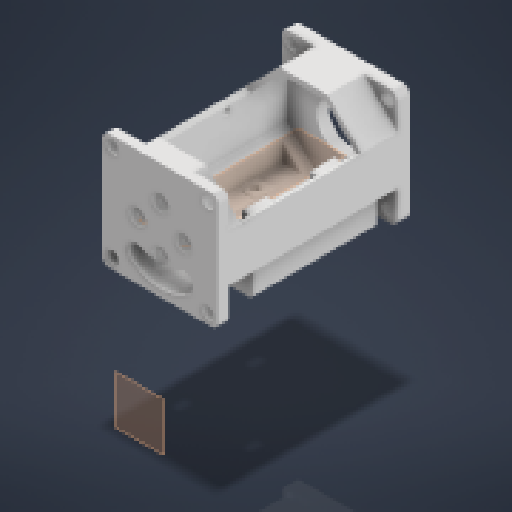
# Autodesk Inventor part: КорпусЕСК
Saved by Autodesk Inventor 2026 (Build 300175000, 175)
## iProperties
Created: 2025-08-20
Part Number: КорпусЕСК
Material: Типовые
Document SubType Name: Modeling
Designer: seraf
Density: 1 g/cm^3
Appearance: По умолчанию
Author: seraf
Autodesk Inventor part; units mm, degrees
ref_plane "YZ Plane" through (0, 0, 0) normal (1, 0, 0) x (0, 1, 0)
ref_plane "XZ Plane" through (0, 0, 0) normal (0, 1, 0) x (-1, 0, 0)
ref_plane "РабПлоскость1" through (0, 0, 25.75) normal (0, 0, 1) x (1, 0, 0)
sketch "Эскиз1" plane through (0, 0, 25.75) normal (0, 0, 1) x (1, 0, 0)
  circle A0 centre (30.5216, 91.6095) radius 2.5 projected
  circle A1 centre (10.7206, 81.3105) radius 1.5 projected
  circle A2 centre (1.2206, 71.8105) radius 1.5 projected
  circle A3 centre (-9.0784, 52.0095) radius 2.5 projected
  circle A4 centre (10.7206, 62.3105) radius 1.5 projected
  circle A5 centre (30.5216, 52.0095) radius 2.5 projected
  circle A6 centre (-9.0784, 91.6095) radius 2.5 projected
  circle A7 centre (20.2206, 71.8105) radius 1.5 projected
  arc A8 (34.7206, 92.8105) -> (31.7206, 95.8105) centre (31.7206, 92.8105) ccw projected
  line L0 (34.7206, 50.8105) -> (34.7206, 92.8105) projected
  arc A9 (31.7206, 47.8105) -> (34.7206, 50.8105) centre (31.7206, 50.8105) ccw projected
  line L1 (-10.2794, 47.8105) -> (31.7206, 47.8105) projected
  arc A10 (-13.2794, 50.8105) -> (-10.2794, 47.8105) centre (-10.2794, 50.8105) ccw projected
  line L2 (-13.2794, 92.8105) -> (-13.2794, 50.8105) projected
  arc A11 (-10.2794, 95.8105) -> (-13.2794, 92.8105) centre (-10.2794, 92.8105) ccw projected
  line L3 (31.7206, 95.8105) -> (-10.2794, 95.8105) projected
  arc A12 (-0.1228, 54.4431) -> (21.5639, 54.4431) centre (10.7206, 68.8105) ccw projected
  arc A13 (21.5639, 54.4431) -> (19.9477, 62.2015) centre (20.2206, 58.2108) ccw projected
  arc A14 (1.4934, 62.2015) -> (19.9477, 62.2015) centre (10.7206, 78.8105) ccw projected
  arc A15 (1.4934, 62.2015) -> (-0.1228, 54.4431) centre (1.2206, 58.2108) ccw projected
  point P0 (0, 0)
extrude "Выдавливание1" add sketch "Эскиз1" along normal blind 2
chamfer "Фаска1" distance 2 angle 45 4 edges at (9.2206, 62.3105, 27.75) (18.7206, 71.8105, 27.75) (9.2206, 81.3105, 27.75) (-0.2794, 71.8105, 27.75)
sketch "Эскиз2" plane through (0, 0, 25.75) normal (0, 0, -1) x (-1, 0, 0)
  line L0 (-31.7206, 95.8105) -> (10.2794, 95.8105) projected
  arc A0 (-31.7206, 95.8105) -> (-34.7206, 92.8105) centre (-31.7206, 92.8105) ccw projected
  line L1 (-34.7206, 50.8105) -> (-34.7206, 92.8105) projected
  arc A1 (-34.7206, 50.8105) -> (-31.7206, 47.8105) centre (-31.7206, 50.8105) ccw projected
  line L2 (10.2794, 47.8105) -> (-31.7206, 47.8105) projected
  arc A2 (10.2794, 47.8105) -> (13.2794, 50.8105) centre (10.2794, 50.8105) ccw projected
  line L3 (13.2794, 92.8105) -> (13.2794, 50.8105) projected
  arc A3 (13.2794, 92.8105) -> (10.2794, 95.8105) centre (10.2794, 92.8105) ccw projected
  circle A4 centre (-10.7206, 81.3105) radius 1.5 construction
  circle A5 centre (-1.2206, 71.8105) radius 1.5 construction
  circle A6 centre (-20.2206, 71.8105) radius 1.5 construction
  arc A7 (-19.9477, 62.2015) -> (-1.4934, 62.2015) centre (-10.7206, 78.8105) ccw projected
  arc A8 (0.1228, 54.4431) -> (-1.4934, 62.2015) centre (-1.2206, 58.2108) ccw projected
  arc A9 (-21.5639, 54.4431) -> (0.1228, 54.4431) centre (-10.7206, 68.8105) ccw projected
  arc A10 (-19.9477, 62.2015) -> (-21.5639, 54.4431) centre (-20.2206, 58.2108) ccw projected
  circle A11 centre (9.0784, 91.6095) radius 2.5 projected
  circle A12 centre (-30.5216, 52.0095) radius 2.5 projected
  circle A13 centre (-10.7206, 62.3105) radius 1.5 construction
  circle A14 centre (9.0784, 52.0095) radius 2.5 projected
  circle A15 centre (-30.5216, 91.6095) radius 2.5 projected
  point P0 (0, 0)
extrude "Выдавливание2" add sketch "Эскиз2" along normal blind 2
sketch "Эскиз3" plane through (0, 0, 23.75) normal (0, 0, -1) x (-1, 0, 0)
  line L0 (-31.7206, 47.8105) -> (10.2794, 47.8105) construction
  arc A0 (10.2794, 47.8105) -> (13.2794, 50.8105) centre (10.2794, 50.8105) ccw construction
  line L1 (13.2794, 50.8105) -> (13.2794, 92.8105) construction
  arc A1 (13.2794, 92.8105) -> (10.2794, 95.8105) centre (10.2794, 92.8105) ccw construction
  line L2 (10.2794, 95.8105) -> (-31.7206, 95.8105) construction
  arc A2 (-31.7206, 95.8105) -> (-34.7206, 92.8105) centre (-31.7206, 92.8105) ccw construction
  line L3 (-34.7206, 92.8105) -> (-34.7206, 50.8105) construction
  arc A3 (-34.7206, 50.8105) -> (-31.7206, 47.8105) centre (-31.7206, 50.8105) ccw construction
  circle A4 centre (-30.5216, 91.6095) radius 2.5 construction
  circle A5 centre (9.0784, 52.0095) radius 2.5 construction
  circle A6 centre (-30.5216, 52.0095) radius 2.5 construction
  circle A7 centre (9.0784, 91.6095) radius 2.5 construction
  arc A8 (-19.9477, 62.2015) -> (-21.5639, 54.4431) centre (-20.2206, 58.2108) ccw construction
  arc A9 (-19.9477, 62.2015) -> (-1.4934, 62.2015) centre (-10.7206, 78.8105) ccw construction
  arc A10 (0.1228, 54.4431) -> (-1.4934, 62.2015) centre (-1.2206, 58.2108) ccw construction
  arc A11 (-21.5639, 54.4431) -> (0.1228, 54.4431) centre (-10.7206, 68.8105) ccw construction
  line L4 (-34.7206, 71.8105) -> (-34.7206, 81.8105)
  line L5 (-34.7206, 81.8105) -> (-20.7206, 95.8105)
  line L6 (-20.7206, 95.8105) -> (-0.7206, 95.8105)
  line L7 (-0.7206, 95.8105) -> (13.2794, 81.8105)
  line L8 (13.2794, 81.8105) -> (13.2794, 71.8105)
  line L9 (-34.7206, 71.8105) -> (13.2794, 71.8105)
  line L10 (13.2794, 92.8105) -> (13.2794, 50.8105) construction
  arc A12 (10.2794, 47.8105) -> (13.2794, 50.8105) centre (10.2794, 50.8105) ccw construction
  line L11 (10.2794, 47.8105) -> (-31.7206, 47.8105) construction
  arc A13 (-34.7206, 50.8105) -> (-31.7206, 47.8105) centre (-31.7206, 50.8105) ccw construction
  line L12 (-34.7206, 50.8105) -> (-34.7206, 92.8105) construction
  circle A14 centre (-30.5216, 52.0115) radius 2.5 construction
  circle A15 centre (9.0784, 52.0115) radius 2.5 construction
  line L13 (-34.7206, 71.8105) -> (-34.7206, 61.8105)
  line L14 (-34.7206, 61.8105) -> (-20.7206, 47.8105)
  line L15 (-20.7206, 47.8105) -> (-0.7206, 47.8105)
  line L16 (-0.7206, 47.8105) -> (13.2794, 61.8105)
  line L17 (13.2794, 61.8105) -> (13.2794, 71.8105)
  line L18 (-1.7206, 50.0826) -> (-19.7206, 50.0826)
  line L19 (-19.7206, 50.0826) -> (-32.4485, 62.8105)
  line L20 (-32.4485, 62.8105) -> (-32.4485, 80.8105)
  line L21 (-32.4485, 80.8105) -> (-19.7206, 93.5384)
  line L22 (-19.7206, 93.5384) -> (-1.7206, 93.5384)
  line L23 (-1.7206, 93.5384) -> (11.0074, 80.8105)
  line L24 (11.0074, 80.8105) -> (11.0074, 62.8105)
  line L25 (11.0074, 62.8105) -> (-1.7206, 50.0826)
  point P0 (0, 0)
  point P1 (-10.7206, 64.8105)
  point P2 (-10.7206, 71.8105)
  dimension "d8" = 20
  dimension "d9" = 1
  constraints: 44 end point, 13 symmetric about line, 8 point on line, 4 centre point, 4 point on circle, 3 midpoint, 2 equal length, 2 perpendicular, 1 horizontal, 21 other
  measures "d8" distance of L5.end L6.end
  measures "d9" horizontal distance of L16.start L18.start
extrude "Выдавливание3" add sketch "Эскиз3" along normal blind 5 contours L4 L5 L6 L7 L8 L9 L24 L23 L22 L21 L20 | L9 L20 L19 L18 L25 L24 L17 L16 L15 L14 L13
sketch "Эскиз4" plane through (0, 0, 18.75) normal (0, 0, -1) x (-1, 0, 0)
  line L0 (-34.7206, 61.8105) -> (-20.7206, 47.8105) projected
  line L1 (-20.7206, 47.8105) -> (-0.7206, 47.8105) projected
  line L2 (-0.7206, 47.8105) -> (13.2794, 61.8105) projected
  line L3 (13.2794, 61.8105) -> (13.2794, 81.8105) projected
  line L4 (13.2794, 81.8105) -> (-0.7206, 95.8105) construction
  line L5 (-0.7206, 95.8105) -> (-20.7206, 95.8105) construction
  line L6 (-20.7206, 95.8105) -> (-34.7206, 81.8105) construction
  line L7 (-34.7206, 81.8105) -> (-34.7206, 61.8105) projected
  line L8 (-32.4485, 62.8105) -> (-32.4485, 80.8105) projected
  line L9 (-32.4485, 80.8105) -> (-19.7206, 93.5384) construction
  line L10 (-19.7206, 93.5384) -> (-1.7206, 93.5384) construction
  line L11 (-1.7206, 93.5384) -> (11.0074, 80.8105) construction
  line L12 (11.0074, 80.8105) -> (11.0074, 62.8105) projected
  line L13 (11.0074, 62.8105) -> (-1.7206, 50.0826) projected
  line L14 (-1.7206, 50.0826) -> (-19.7206, 50.0826) projected
  line L15 (-19.7206, 50.0826) -> (-32.4485, 62.8105) projected
  line L16 (-34.7206, 81.8105) -> (-32.4485, 80.8105)
  line L17 (13.2794, 81.8105) -> (11.0074, 80.8105)
  point P0 (0, 0)
  constraints: 4 end point
extrude "Выдавливание4" add sketch "Эскиз4" along normal blind 50
sketch "Эскиз5" plane through (0, 0, -31.25) normal (0, 0, -1) x (-1, 0, 0)
  line L0 (-34.7206, 61.8105) -> (-20.7206, 47.8105) projected
  line L1 (-20.7206, 47.8105) -> (-0.7206, 47.8105) projected
  line L2 (-0.7206, 47.8105) -> (13.2794, 61.8105) projected
  line L3 (13.2794, 61.8105) -> (13.2794, 81.8105) projected
  line L4 (13.2794, 81.8105) -> (11.0074, 80.8105) construction
  line L5 (11.0074, 80.8105) -> (11.0074, 62.8105) projected
  line L6 (11.0074, 62.8105) -> (-1.7206, 50.0826) projected
  line L7 (-1.7206, 50.0826) -> (-19.7206, 50.0826) projected
  line L8 (-19.7206, 50.0826) -> (-32.4485, 62.8105) projected
  line L9 (-32.4485, 62.8105) -> (-32.4485, 80.8105) projected
  line L10 (-32.4485, 80.8105) -> (-34.7206, 81.8105) construction
  line L11 (-34.7206, 81.8105) -> (-34.7206, 61.8105) projected
  line L12 (11.0074, 80.8105) -> (13.2794, 81.8105) construction
  line L13 (13.2794, 81.8105) -> (-0.7206, 95.8105) projected
  line L14 (-0.7206, 95.8105) -> (-20.7206, 95.8105) projected
  line L15 (-20.7206, 95.8105) -> (-34.7206, 81.8105) projected
  line L16 (-34.7206, 81.8105) -> (-32.4485, 80.8105) construction
  line L17 (-32.4485, 80.8105) -> (-19.7206, 93.5384) projected
  line L18 (-19.7206, 93.5384) -> (-1.7206, 93.5384) projected
  line L19 (-1.7206, 93.5384) -> (11.0074, 80.8105) projected
  point P0 (0, 0)
extrude "Выдавливание5" add sketch "Эскиз5" along normal blind 15
sketch "Эскиз6" plane through (0, 0, -46.25) normal (0, 0, -1) x (-1, 0, 0)
  circle A0 centre (-10.7206, 81.3105) radius 3.5 construction
  circle A1 centre (-30.5216, 91.6095) radius 2.5 projected
  circle A2 centre (9.0784, 52.0095) radius 2.5 projected
  circle A3 centre (-30.5216, 52.0095) radius 2.5 projected
  circle A4 centre (9.0784, 91.6095) radius 2.5 projected
  line L0 (-31.7206, 95.8105) -> (10.2794, 95.8105) projected
  arc A5 (13.2794, 92.8105) -> (10.2794, 95.8105) centre (10.2794, 92.8105) ccw projected
  line L1 (13.2794, 92.8105) -> (13.2794, 50.8105) projected
  arc A6 (10.2794, 47.8105) -> (13.2794, 50.8105) centre (10.2794, 50.8105) ccw projected
  line L2 (10.2794, 47.8105) -> (-31.7206, 47.8105) projected
  arc A7 (-34.7206, 50.8105) -> (-31.7206, 47.8105) centre (-31.7206, 50.8105) ccw projected
  line L3 (-34.7206, 50.8105) -> (-34.7206, 92.8105) projected
  arc A8 (-31.7206, 95.8105) -> (-34.7206, 92.8105) centre (-31.7206, 92.8105) ccw projected
  arc A9 (-8.0984, 59.9923) -> (-13.3428, 59.9923) centre (-10.7206, 62.3105) ccw construction
  arc A10 (-19.9477, 62.2015) -> (-13.3428, 59.9923) centre (-10.7206, 78.8105) ccw construction
  arc A11 (-19.9477, 62.2015) -> (-21.5639, 54.4431) centre (-20.2206, 58.2108) ccw construction
  arc A12 (-21.5639, 54.4431) -> (0.1228, 54.4431) centre (-10.7206, 68.8105) ccw construction
  arc A13 (0.1228, 54.4431) -> (-1.4934, 62.2015) centre (-1.2206, 58.2108) ccw construction
  arc A14 (-8.0984, 59.9923) -> (-1.4934, 62.2015) centre (-10.7206, 78.8105) ccw construction
  circle A15 centre (-20.2206, 71.8105) radius 3.5 construction
  circle A16 centre (-1.2206, 71.8105) radius 3.5 construction
  circle A17 centre (-10.7206, 71.8105) radius 9.5
  point P0 (0, 0)
  dimension "d16" = 19
  constraints: 2 point on circle, 1 centre point
  measures "d16" diameter of A17
extrude "Выдавливание6" add sketch "Эскиз6" along normal blind 5
ref_plane "РабПлоскость3" through (1.7206, 70.0826, 23.75) normal (0, 1, 0) x (1, 0, 0)
sketch "Эскиз8" plane through (1.7206, 70.0826, 23.75) normal (0, 1, 0) x (1, 0, 0)
  line L0 (30, -4) -> (33, -4) projected
  line L1 (-12, 75) -> (-15, 75) projected
  line L2 (-15, 75) -> (33, 75) construction
  line L3 (33, 75) -> (33, -4) construction
  line L4 (33, -4) -> (-15, -4) construction
  line L5 (-15, -4) -> (-15, 75) construction
  circle A0 centre (23.75, 50) radius 1.5 construction
  line L6 (23.75, 50) -> (23.75, 19.5) construction
  line L7 (23.75, 19.5) -> (-5.75, 19.5) construction
  line L8 (-5.75, 19.5) -> (-5.75, 50) construction
  circle A1 centre (-5.75, 50) radius 1.5
  circle A2 centre (23.75, 19.5) radius 1.5
  circle A3 centre (-5.75, 19.5) radius 1.5
  circle A4 centre (-5.75, 50) radius 4
  circle A5 centre (-5.75, 19.5) radius 4
  circle A6 centre (23.75, 19.5) radius 4
  point P0 (-1.7206, 23.75)
  dimension "d22" = 3
  dimension "d23" = 9.25
  dimension "d24" = 25
  dimension "d25" = 29.5
  dimension "d26" = 30.5
  dimension "d27" = 30.5
  dimension "d28" = 3
  dimension "d29" = 3
  dimension "d30" = 3
  dimension "d31" = 8
  dimension "d32" = 8
  dimension "d33" = 8
  constraints: 14 end point, 7 centre point, 6 coincident, 2 parallel, 2 perpendicular, 2 vertical, 1 horizontal
  measures "d22" diameter of A0
  measures "d23" distance from line of L3 L6.start
  measures "d24" distance from line of L2 L6.start
  measures "d25" distance of L6.end L7.end
  measures "d26" distance of L7.end L8.end
  measures "d27" distance of L6.start L6.end
  measures "d28" diameter of A1
  measures "d29" diameter of A2
  measures "d30" diameter of A3
  measures "d31" diameter of A4
  measures "d32" diameter of A5
  measures "d33" diameter of A6
extrude "Выдавливание7" add sketch "Эскиз8" against normal up to surface contours A4 | A5 surface through (-11.0074, 62.8105, 23.75) normal (0.7071068, 0.7071068, 0)
sketch "Эскиз11" plane through (-4.0294, 70.0826, 4.25) normal (0, 1, 0) x (1, 0, 0)
  circle A0 centre (0, 0) radius 4 projected
  circle A1 centre (0, 0) radius 1.5 projected
  line L0 (-6.25, 55.5) -> (35.75, 55.5) construction
  line L1 (14.75, 55.5) -> (14.75, -23.5)
  line L2 (11.25, -23.5) -> (18.25, -23.5) projected
  circle A2 centre (29.5, 0) radius 4
  circle A3 centre (29.5, 0) radius 1.5
  point P0 (4.0294, 4.25)
  point P1 (17.3722, -23.5)
  point P2 (12.1278, -23.5)
  constraints: 2 centre point, 2 end point, 2 midpoint, 2 symmetric about line, 2 other
extrude "Выдавливание9" add sketch "Эскиз11" against normal up to surface contours A2 surface through (19.7206, 50.0826, 23.75) normal (-0.7071068, 0.7071068, 0)
sketch "Эскиз12" plane through (-10.2794, 47.8105, 27.75) normal (0, -1, 0) x (1, 0, 0)
  circle A0 centre (6.25, -23.5) radius 4 construction
  circle A1 centre (6.25, -23.5) radius 1.5 construction
  circle A2 centre (6.25, -54) radius 4 construction
  circle A3 centre (6.25, -54) radius 1.5 construction
  circle A4 centre (35.75, -23.5) radius 4 construction
  circle A5 centre (35.75, -23.5) radius 1.5 construction
  line L0 (40.75, -18.5) -> (1.25, -18.5)
  line L1 (1.25, -18.5) -> (1.25, -59)
  line L2 (1.25, -59) -> (40.75, -59)
  line L3 (40.75, -59) -> (40.75, -18.5)
  point P0 (10.2794, -27.75)
  dimension "d40" = 5
  dimension "d41" = 5
  dimension "d42" = 5
  dimension "d43" = 5
  constraints: 8 end point, 2 parallel, 1 horizontal, 1 perpendicular
  measures "d40" horizontal distance of L1.end A2.centre
  measures "d41" horizontal distance of L1.end A2.centre
  measures "d42" distance from line of L0 A5.centre
  measures "d43" distance from line of L3 A4.centre
extrude "Выдавливание10" add sketch "Эскиз12" against normal up to surface (2.2721 mm away)
sketch "Эскиз13" plane through (22.9926, 50.0826, 9.25) normal (0, 1, 0) x (1, 0, 0)
  line L0 (0, 0) -> (0, 40.5) projected
  line L1 (7.4779, 0) -> (0, 0) projected
  line L2 (7.4779, 40.5) -> (7.4779, 0) projected
  line L3 (0, 40.5) -> (7.4779, 40.5) projected
  line L4 (-24.5442, 40.5) -> (-24.5442, 0) projected
  line L5 (-32.0221, 40.5) -> (-24.5442, 40.5) projected
  line L6 (-32.0221, 0) -> (-32.0221, 40.5) projected
  line L7 (-24.5442, 0) -> (-32.0221, 0) projected
  point P0 (-22.9926, 9.25)
extrude "Выдавливание11" add sketch "Эскиз13" along normal up to surface contours L0 L3 L2 L1 surface through (19.7206, 50.0826, 23.75) normal (-0.7071068, 0.7071068, 0)
sketch "Эскиз14" plane through (-9.0294, 50.0826, -31.25) normal (0, 1, 0) x (1, 0, 0)
  line L0 (7.4779, 0) -> (7.4779, -40.5) projected
  line L1 (0, 0) -> (7.4779, 0) projected
  line L2 (0, -40.5) -> (0, 0) projected
  line L3 (7.4779, -40.5) -> (0, -40.5) projected
  point P0 (9.0294, -31.25)
extrude "Выдавливание12" add sketch "Эскиз14" along normal up to surface surface through (-11.0074, 62.8105, 23.75) normal (0.7071068, 0.7071068, 0)
chamfer "Фаска2" distance 1 angle 45 2 edges at (-9.0294, 47.8105, -11) (30.4706, 47.8105, -11)
sketch "Эскиз15" plane through (25.4706, 70.0826, 4.25) normal (0, 1, 0) x (1, 0, 0)
  circle A0 centre (0, 0) radius 4 construction
  circle A1 centre (0, 0) radius 1.5 construction
  circle A2 centre (-29.5, 30.5) radius 4 projected
  circle A3 centre (-29.5, 30.5) radius 1.5 projected
  circle A4 centre (-29.5, 0) radius 4 construction
  circle A5 centre (-29.5, 0) radius 1.5 construction
  line L0 (-33.5, -4) -> (4, -4)
  line L1 (4, -4) -> (4, 34.5)
  line L2 (4, 34.5) -> (-33.5, 34.5)
  line L3 (-33.5, 34.5) -> (-33.5, -4)
  circle A6 centre (-29.5, 0) radius 4 projected
  circle A7 centre (0, 0) radius 4 projected
  point P0 (-25.4706, 4.25)
  point P1 (-33.5, 0)
  point P2 (-29.5, -4)
  point P3 (0, -4)
  point P4 (4, 0)
  point P5 (-29.5, 34.5)
  point P6 (-33.5, 30.5)
  constraints: 8 end point, 4 tangent, 2 parallel, 1 horizontal, 1 perpendicular
extrude "Выдавливание13" cut sketch "Эскиз15" against normal blind 18 contours A2 L2 L1 A7 L0 A6 L3 | A2 L3 L2 | A3
sketch "Эскиз16" plane through (-4.0294, 70.0826, -26.25) normal (0, 1, 0) x (1, 0, 0)
  circle A0 centre (0, 0) radius 4 projected
  circle A1 centre (0, 0) radius 1.5 projected
  circle A2 centre (0, -30.5) radius 4 projected
  circle A3 centre (0, -30.5) radius 1.5 projected
  circle A4 centre (29.5, -30.5) radius 4 projected
  circle A5 centre (29.5, -30.5) radius 1.5 projected
  point P0 (4.0294, -26.25)
extrude "Выдавливание14" cut sketch "Эскиз16" against normal blind 18 contours A1 | A3 | A5
sketch "Эскиз17" plane through (25.4706, 70.0826, 4.25) normal (0, 1, 0) x (1, 0, 0)
  circle A0 centre (0, 0) radius 4 projected
  circle A1 centre (0, 0) radius 1.5 projected
  circle A2 centre (-29.5, 0) radius 4 projected
  circle A3 centre (-29.5, 0) radius 1.5 projected
  circle A4 centre (-29.5, 30.5) radius 4 projected
  circle A5 centre (-29.5, 30.5) radius 1.5 projected
  point P0 (-25.4706, 4.25)
extrude "Выдавливание15" cut sketch "Эскиз17" against normal blind 17.5
sketch "Эскиз18" plane through (25.4706, 52.0826, 4.25) normal (0, 1, 0) x (1, 0, 0)
  arc A0 (-29.5, 34.5) -> (-33.5, 30.5) centre (-29.5, 30.5) ccw projected
  line L0 (-33.5, 34.5) -> (-29.5, 34.5) projected
  line L1 (-33.5, 30.5) -> (-33.5, 34.5) projected
  line L2 (-3.75, 1.3919) -> (-3.75, 34.5) projected
  arc A1 (4, 0) -> (-3.75, 1.3919) centre (0, 0) ccw projected
  line L3 (4, 34.5) -> (4, 0) projected
  line L4 (-3.75, 34.5) -> (4, 34.5) projected
  line L5 (4, 34.5) -> (-33.5, 34.5)
  line L6 (-33.5, 34.5) -> (-33.5, 46.5)
  line L7 (-33.5, 46.5) -> (4, 46.5)
  line L8 (4, 46.5) -> (4, 34.5)
  point P0 (-25.4706, 4.25)
  dimension "d60" = 12
  constraints: 8 end point, 2 parallel, 1 horizontal, 1 perpendicular
  measures "d60" distance of L5.end L6.end
extrude "Выдавливание16" cut sketch "Эскиз18" along normal blind 15 contours L0 L6 L7 L8 L4 L5
sketch "Эскиз19" plane through (29.4706, 47.8105, -31.25) normal (0, 0, -1) x (-1, 0, 0)
  line L0 (37.5, 4.2721) -> (33.0221, 4.2721) projected
  line L1 (28.75, 0) -> (33.0221, 4.2721) projected
  line L2 (37.5, 0) -> (28.75, 0) projected
  line L3 (38.5, 1) -> (37.5, 0) projected
  line L4 (38.5, 1) -> (38.5, 9.75) projected
  line L5 (37.5, 8.75) -> (38.5, 9.75) projected
  line L6 (37.5, 8.75) -> (37.5, 4.2721) projected
  line L7 (4.4779, 4.2721) -> (0, 4.2721) projected
  line L8 (0, 4.2721) -> (0, 8.75) projected
  line L9 (-1, 9.75) -> (0, 8.75) projected
  line L10 (-1, 1) -> (-1, 9.75) projected
  line L11 (0, 0) -> (-1, 1) projected
  line L12 (8.75, 0) -> (0, 0) projected
  line L13 (4.4779, 4.2721) -> (8.75, 0) projected
  point P0 (29.4706, -47.8105)
extrude "Выдавливание17" add sketch "Эскиз19" along normal up to surface (11 mm away)
sketch "Эскиз20" plane through (-3.5515, 52.0826, -42.25) normal (0, 0, 1) x (1, 0, 0)
  line L0 (3.2721, 0) -> (0, 0) projected
  line L1 (-4.4779, 0) -> (3.2721, 0)
  line L2 (3.2721, 0) -> (-4.4779, 7.75)
  line L3 (-4.4779, 7.75) -> (3.2721, 0) projected
  line L4 (-4.4779, 7.75) -> (-4.4779, 0)
  line L5 (28.5442, 0) -> (25.2721, 0) projected
  line L6 (25.2721, 0) -> (33.0221, 7.75) projected
  line L7 (25.2721, 0) -> (33.0221, 7.75)
  line L8 (33.0221, 7.75) -> (33.0221, 0)
  line L9 (33.0221, 0) -> (25.2721, 0)
  point P0 (3.5515, -52.0826)
  constraints: 12 end point, 2 collinear, 2 perpendicular, 1 horizontal
extrude "Выдавливание18" add sketch "Эскиз20" along normal blind 1
sketch "Эскиз21" plane through (-4.0294, 52.0826, -26.25) normal (0, 1, 0) x (1, 0, 0)
  circle A0 centre (0, -30.5) radius 1.5 projected
  circle A1 centre (29.5, -30.5) radius 1.5 projected
  circle A2 centre (29.5, -30.5) radius 1.5 projected
  circle A3 centre (0, 0) radius 1.5 projected
  point P0 (4.0294, -26.25)
extrude "Выдавливание19" cut sketch "Эскиз21" against normal through all
sketch "Эскиз22" plane through (-13.2794, 50.8105, 27.75) normal (-1, 0, 0) x (0, 0, 1)
  line L0 (-9, 31) -> (-59, 31) construction
  circle A0 centre (-49, 28.1085) radius 1.5
  circle A1 centre (-19, 28.1085) radius 1.5
  point P0 (-27.75, -50.8105)
  dimension "d69" = 3
  dimension "d70" = 3
  dimension "d72" = 10
  dimension "d73" = 10
  constraints: 2 centre point, 1 horizontal alignment
  measures "d69" diameter of A0
  measures "d70" diameter of A1
  measures "d72" horizontal distance of L0.end A0.centre
  measures "d73" horizontal distance of L0.start A1.centre
extrude "Выдавливание20" cut sketch "Эскиз22" against normal blind 3.25
sketch "Эскиз23" plane through (32.4485, 62.8105, 23.75) normal (-1, 0, 0) x (0, 0, 1)
  line L0 (-5, 19) -> (-55, 19) construction
  line L1 (-5, 18) -> (-55, 18) construction
  line L2 (-49, 18) -> (-39, 18)
  line L3 (-39, 18) -> (-39, 13)
  line L4 (-39, 13) -> (-49, 13)
  line L5 (-49, 13) -> (-49, 18)
  line L6 (-48.2, 17.2) -> (-39.8, 17.2)
  line L7 (-39.8, 17.2) -> (-39.8, 13.8)
  line L8 (-39.8, 13.8) -> (-48.2, 13.8)
  line L9 (-48.2, 13.8) -> (-48.2, 17.2)
  line L10 (-30, 19) -> (-30, 11.3763)
  line L11 (-11, 18) -> (-21, 18)
  line L12 (-21, 18) -> (-21, 13)
  line L13 (-21, 13) -> (-11, 13)
  line L14 (-11, 13) -> (-11, 18)
  line L15 (-11.8, 17.2) -> (-20.2, 17.2)
  line L16 (-20.2, 17.2) -> (-20.2, 13.8)
  line L17 (-20.2, 13.8) -> (-11.8, 13.8)
  line L18 (-11.8, 13.8) -> (-11.8, 17.2)
  point P0 (-23.75, -62.8105)
  dimension "d76" = 10
  dimension "d77" = 5
  dimension "d80" = 6
  dimension "d82" = 0.8
  dimension "d83" = 0.8
  dimension "d84" = 0.8
  dimension "d85" = 0.8
  constraints: 34 end point, 8 symmetric about line, 4 parallel, 2 horizontal, 2 perpendicular, 1 midpoint, 1 point on line, 1 vertical
  measures "d76" distance of L3.end L4.end
  measures "d77" distance of L2.end L3.end
  measures "d80" distance of L1.end L2.start
  measures "d82" horizontal distance of L2.end L6.end
  measures "d83" distance from line of L3 L6.end
  measures "d84" horizontal distance of L4.end L8.end
  measures "d85" distance from line of L5 L8.end
extrude "Выдавливание21" add sketch "Эскиз23" along normal blind 3
chamfer "Фаска3" distance 3 angle 45 2 edges at (32.4485, 75.8105, -20.25) (32.4485, 75.8105, 7.75)
